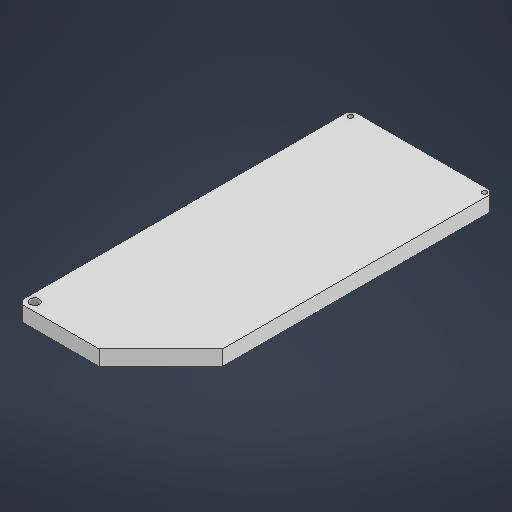
# Autodesk Inventor part: Top
Saved by Autodesk Inventor 2026.1 (Build 301233020, 233B)
## iProperties
Created: 2026-05-28
Part Number: Top
Material: Generic
Document SubType Name: Modeling
Designer: jcla0
Density: 1 g/cm^3
Appearance: Default
Author: jcla0
Autodesk Inventor part; units mm, degrees
ref_plane "YZ Plane" through (0, 0, 0) normal (1, 0, 0) x (0, 1, 0)
ref_plane "XZ Plane" through (0, 0, 0) normal (0, 1, 0) x (-1, 0, 0)
sketch "Sketch1" plane through (0, 0, 0) normal (0, 1, 0) x (-1, 0, 0)
  line L0 (21.5102, 17.7267) -> (21.5102, -43.9733)
  line L1 (21.5102, -43.9733) -> (19.1102, -46.7733)
  line L2 (19.1102, -46.7733) -> (-5.4898, -46.7733)
  line L3 (-5.4898, -46.7733) -> (-7.4898, -44.7733)
  line L4 (-7.4898, -44.7733) -> (-7.4898, 9.2267)
  line L5 (-7.4898, 9.2267) -> (5.5102, 22.2267)
  line L6 (5.5102, 22.2267) -> (17.0102, 22.2267)
  line L7 (17.0102, 22.2267) -> (21.5102, 17.7267)
  line L8 (22.0102, 21.7267) -> (22.0102, -46.2733)
  line L9 (22.0102, -46.2733) -> (21.0102, -47.2733)
  line L10 (21.0102, -47.2733) -> (-6.9898, -47.2733)
  line L11 (-6.9898, -47.2733) -> (-7.9898, -46.2733)
  line L12 (-7.9898, -46.2733) -> (-7.9898, 9.7267)
  line L13 (-7.9898, 9.7267) -> (5.0102, 22.7267)
  line L14 (5.0102, 22.7267) -> (21.0102, 22.7267)
  line L15 (21.0102, 22.7267) -> (22.0102, 21.7267)
  point P0 (0, 0)
  point P1 (14.1019, -14.4492)
  dimension "d0" = 69
  dimension "d1" = 29
  dimension "d2" = 2
  dimension "d3" = 2
  dimension "d4" = 2.8
  dimension "d5" = 2.4
  dimension "d6" = 4.5
  dimension "d7" = 4.5
  dimension "d8" = 13
  dimension "d9" = 13
  dimension "d10" = 70
  dimension "d11" = 30
  dimension "d12" = 1
  dimension "d13" = 1
  dimension "d14" = 1
  dimension "d15" = 1
  dimension "d16" = 1
  dimension "d17" = 1
  dimension "d18" = 13
  dimension "d19" = 13
  dimension "d34" = 0.5
  dimension "d35" = 0.5
  constraints: 32 end point, 4 parallel, 2 perpendicular, 2 vertical
  measures "d0" distance between parallel lines of L2 L6
  measures "d1" distance between parallel lines of L0 L4
  measures "d2" horizontal distance of L2.end L3.end
  measures "d3" horizontal distance of L2.end L3.end
  measures "d4" vertical distance of L1.end L0.end
  measures "d5" horizontal distance of L1.end L0.end
  measures "d6" horizontal distance of L0.start L6.end
  measures "d7" horizontal distance of L0.start L6.end
  measures "d8" horizontal distance of L4.end L5.end
  measures "d9" horizontal distance of L4.end L5.end
  measures "d10" distance between parallel lines of L10 L14
  measures "d11" distance between parallel lines of L8 L12
  measures "d12" horizontal distance of L10.end L11.end
  measures "d13" horizontal distance of L10.end L11.end
  measures "d14" horizontal distance of L9.end L8.end
  measures "d15" horizontal distance of L9.end L8.end
  measures "d16" horizontal distance of L8.start L14.end
  measures "d17" horizontal distance of L8.start L14.end
  measures "d18" horizontal distance of L12.end L13.end
  measures "d19" horizontal distance of L12.end L13.end
  measures "d34" distance between parallel lines of L14 L6
  measures "d35" distance between parallel lines of L12 L4
extrude "Extrusion1" add sketch "Sketch1" along normal blind 3.175 contours L0 L1 L2 L3 L4 L5 L6 L7 | L8 L9 L10 L11 L12 L13 L14 L15
ref_plane "Work Plane3" through (0, 0.5, 0) normal (0, 1, 0) x (1, 0, 0)
sketch "Sketch5" plane through (0, 0.5, 0) normal (0, 1, 0) x (1, 0, 0)
  circle A0 centre (-20.3864, -20.9025) radius 1
  circle A1 centre (-20.8742, 46.0372) radius 0.5
  circle A2 centre (7.0371, 46.2575) radius 0.5
  point P0 (0, 0)
  dimension "d55" = 2
  dimension "d56" = 1
  dimension "d57" = 1
  constraints: 3 centre point
  measures "d55" diameter of A0
  measures "d56" diameter of A1
  measures "d57" diameter of A2
extrude "Extrusion6" cut sketch "Sketch5" along normal blind 3.175 and the other way blind 1.6002
equation "\"d9\" = d8"
equation "\"d19\" = d18"
body "Solid1"
